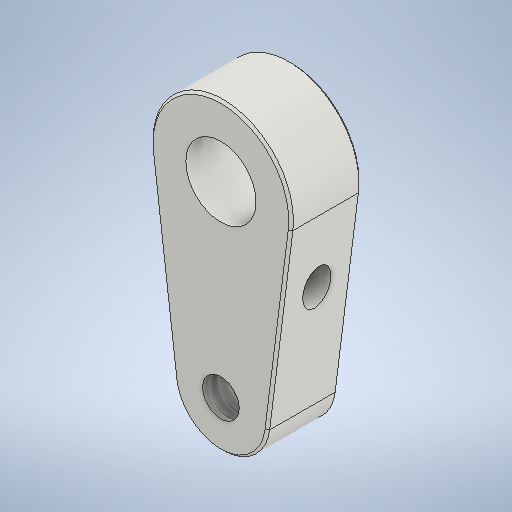
# Autodesk Inventor part: 27 - Valve Level
Saved by Autodesk Inventor 2025.2 (Build 292293000, 293)
## iProperties
Created: 2025-07-17
Part Number: 27 - Valve Level
Material: Steel AISI 1020 108 ANLD
Document SubType Name: Modeling
Designer: bless
Density: 7.87 g/cm^3
Appearance: Steel
Author: bless
Autodesk Inventor part; units mm, degrees
ref_plane "YZ Plane" through (0, 0, 0) normal (1, 0, 0) x (0, 1, 0)
ref_plane "XZ Plane" through (0, 0, 0) normal (0, 1, 0) x (-1, 0, 0)
sketch "Sketch1" plane through (0, 0, 0) normal (0, 0, 1) x (1, 0, 0)
  arc A0 (-1.9843, -0.25) -> (1.9843, -0.25) centre (0, 0) ccw
  arc A1 (2.9765, 7.625) -> (-2.9765, 7.625) centre (0, 8) ccw
  line L0 (2.9765, 7.625) -> (1.9843, -0.25)
  line L1 (-2.9765, 7.625) -> (-1.9843, -0.25)
  circle A2 centre (0, 8) radius 1.5
  dimension "d0" = 3
  dimension "d1" = 2
  dimension "d2" = 8
  dimension "d3" = 3
  constraints: 6 point on circle, 4 end point, 4 tangent, 3 centre point, 2 coincident, 2 point on line, 1 vertical alignment
  measures "d0" radius of A1
  measures "d1" radius of A0
  measures "d2" distance of point (0, 0) A1.centre
  measures "d3" diameter of A2
extrude "Extrusion1" add sketch "Sketch1" along normal blind 3
sketch "Sketch2" plane through (0, 0, 3) normal (0, 0, 1) x (1, 0, 0)
  arc A0 (-1.9843, -0.25) -> (1.9843, -0.25) centre (0, 0) ccw projected
hole "Hole1" at (0, 0, 3) direction (0, 0, -1) diameter 1.567 end through all thread size "M2x0.4" class "6H" standard "ANSI Metric M Profile"
ref_plane "Work Plane2" through (1.7501, 9.2049, 0) normal (0.6132, -0.7899, 0) x (0, 0, 1)
ref_plane "Work Plane1" through (2.9765, 7.625, 0) normal (0.6132, -0.7899, 0) x (0, 0, 1)
sketch "Sketch3" plane through (1.7501, 9.2049, 0) normal (0.6132, -0.7899, 0) x (0, 0, 1)
  line L0 (0, 5.6125) -> (0, 0) projected
  line L1 (0, 0) -> (0, 4.7025) projected
  line L2 (0, 4.7025) -> (3, 4.7025) projected
  line L3 (3, 0) -> (3, 4.7025) projected
  line L4 (0, 0) -> (3, 0) projected
  line L5 (0, -0.8787) -> (3, -0.8787) projected
  point P0 (0, 7.0267)
  point P1 (1.5, 2.1213)
  point P2 (1.5, -0.8787)
  dimension "d15" = 1.5
  dimension "d16" = 3
  constraints: 1 midpoint
  measures "d15" distance from line of L0 point (1.5, 2.121)
  measures "d16" distance of point (1.5, -0.879) point (1.5, 2.121)
hole "Hole2" at (0.0744, 7.9042, 1.5) direction (0.6132, -0.7899, 0) diameter 1.1835 end through all thread size "M1.4x0.3" class "6H" standard "ANSI Metric M Profile"
chamfer "Chamfer1" distance 0.1 angle 45 8 edges at (0, 11, 3) (-2.4804, 3.6875, 3) (0, -2, 3) (2.4804, 3.6875, 3) (2.4804, 3.6875, 0) (0, 11, 0) (-2.4804, 3.6875, 0) (0, -2, 0)
body "Solid1"
